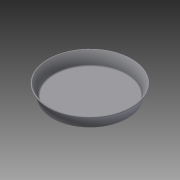
# Autodesk Inventor part: plato1
Saved by Autodesk Inventor 2015 (Build 190159000, 159)
## iProperties
Created: 2016-09-05
Part Number: plato1
Material: Generic
Document SubType Name: Modeling
Designer: Administrator
Density: 1 g/cm^3
Appearance: Default
Author: Administrator
Autodesk Inventor part; units mm, degrees
ref_plane "YZ Plane" through (0, 0, 0) normal (1, 0, 0) x (0, 1, 0)
ref_plane "XZ Plane" through (0, 0, 0) normal (0, 1, 0) x (-1, 0, 0)
ref_plane "XY Plane" through (0, 0, 0) normal (0, 0, 1) x (1, 0, 0)
sketch "Sketch1" plane through (0, 0, 0) normal (1, 0, 0) x (0, 1, 0)
  line L0 (-100.4924, 0) -> (16.7487, 0) projected
  line L1 (0, -4.1746) -> (0, 23.1754) projected
  arc A0 (-56.7738, 1.2743) -> (-63.1144, 17.4194) centre (-83.7437, 0) ccw
  arc A1 (-61.7392, 18.5806) -> (-63.1144, 17.4194) centre (-62.4268, 18) ccw
  arc A2 (-55, 1.8) -> (-61.7392, 18.5806) centre (-83.7437, 0) ccw
  line L2 (-55.4379, 0) -> (0, 0)
  line L3 (-55, 1.8) -> (0, 1.8)
  arc A3 (-56.7738, 1.2743) -> (-55.4379, 0) centre (-55.4379, 1.3374) ccw
  dimension "d0" = 0.9
  dimension "d1" = 55
  dimension "d2" = 1.8
  dimension "d3" = 18
  dimension "d6" = 27
  constraints: 10 point on circle, 4 centre point, 4 end point, 4 tangent, 2 point on line, 1 coincident, 1 collinear, 1 horizontal
  measures "d0" radius of A1
  measures "d1" distance of L3.start L3.end
  measures "d2" distance between parallel lines of L0 L3
  measures "d3" vertical distance of A0.centre A1.centre
  measures "d6" radius of A0
revolve "Revolution1" add sketch "Sketch1" angle 360 about axis through (0, 0, -10) along (0, 0, 1)
fillet "Fillet1" radius 2 1 edges at (0, 55, 1.8)
body "Solid1"
